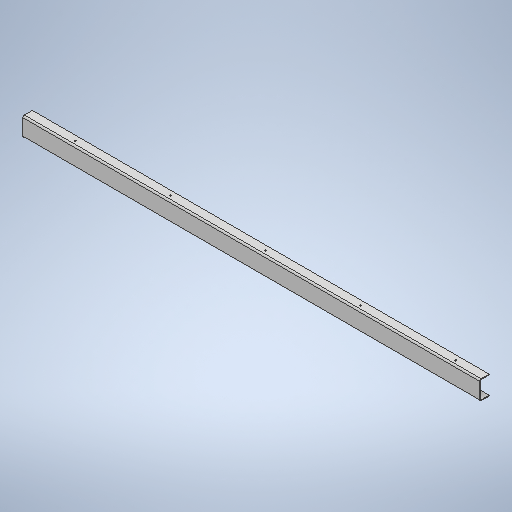
# Autodesk Inventor part: B_Beam
Saved by Autodesk Inventor 2025.2 (Build 292293000, 293)
## iProperties
Created: 2025-04-01
Part Number: B_Beam
Material: Generic
Document SubType Name: Sheet Metal
Designer: Caspe
Density: 1 g/cm^3
Sheet Metal Rule: Default_mm
Appearance: Default
Author: Caspe
Autodesk Inventor part; units mm, degrees
ref_plane "YZ Plane" through (0, 0, 0) normal (1, 0, 0) x (0, 1, 0)
ref_plane "XZ Plane" through (0, 0, 0) normal (0, 1, 0) x (-1, 0, 0)
ref_plane "XY Plane" through (0, 0, 0) normal (0, 0, 1) x (1, 0, 0)
sketch "Sketch2" plane through (0, 0, 0) normal (0, 0, 1) x (-1, 0, 0)
  line L0 (0, 0) -> (-1200, 0)
  line L1 (-1200, 0) -> (-1200, -50)
  line L2 (-1200, -50) -> (0, -50)
  line L3 (0, -50) -> (0, 0)
  dimension "d2" = 1200
  dimension "d3" = 50
  measures "d2" distance of L2.end L1.end
  measures "d3" distance of L1.end L0.end
extrude "Plate1" add sketch "Sketch2" along normal blind 2
sketch "Sketch3" plane through (1200, 48, 2) normal (0, 1, 0) x (-1, 0, 0)
  line L0 (1200, 0) -> (0, 0)
  line L1 (0, 0) -> (0, -25)
  line L2 (0, -25) -> (1200, -25)
  line L3 (1200, -25) -> (1200, 0)
  constraints: 6 end point, 1 horizontal, 1 perpendicular, 1 vertical
edge flange "Flange1" height 25 angle 90 thickness 2 bend radius 2 thickness toward (0, 1, 0) relief straight relief width 2 relief depth 1 corner gap 2 corner form 0 edges at (600, 50, 0) (600, 0, 0) wall of the first edge with corners at (0, 48, 2) (1200, 48, 2) (1200, 48, -23) (0, 48, -23)
bend "Bend1"
corner "Corner1"
sketch "Sketch4" plane through (0, 50, -23) normal (0, 1, 0) x (1, 0, 0)
  circle A0 centre (125, -12.5) radius 2
  line L0 (1200, -25) -> (0, -25) projected
  line L1 (0, -21) -> (0, 0) projected
  circle A1 centre (375, -12.5) radius 2
  circle A2 centre (625, -12.5) radius 2
  circle A3 centre (875, -12.5) radius 2
  circle A4 centre (1125, -12.5) radius 2
  point P0 (0, -23)
  dimension "d15" = 4
  dimension "d16" = 12.5
  dimension "d17" = 125
  dimension "d20" = 250
  constraints: 5 centre point, 1 horizontal, 8 other
  measures "d15" diameter of A0
  measures "d16" distance from line of L0 A0.centre
  measures "d17" distance from line of L1 A0.centre
  measures "d20" distance of A0.centre A1.centre
extrude "Cut1" cut sketch "Sketch4" against normal up to surface (50 mm away)
equation "\"d2\" = B_length"
equation "\"d3\" = B_width"
equation "\"d15\" = rivet_diameter"
equation "\"d16\" = 0.25 * B_width"
equation "\"d17\" = 0.5 * rivet_displacement"
equation "\"d20\" = rivet_displacement"
equation "\"d25\" = Thickness"
equation "\"d4\" = Thickness"
equation "\"d5\" = BendReliefWidth"
equation "\"d6\" = BendReliefDepth"
equation "\"d7\" = MinimumRemnant"
equation "\"d8\" = TransitionRadius"
equation "\"d9\" = 0.5 * B_width"
equation "\"d11\" = BendRadius"
equation "\"d12\" = CornerReliefSize"
equation "\"d13\" = GapSize"
equation "\"d14\" = JacobiRadiusSize"
equation "\"Thickness\" = plate_thickness"
equation "\"BendRadius\" = Thickness"
equation "\"BendReliefWidth\" = Thickness"
equation "\"BendReliefDepth\" = 0.5 * Thickness"
equation "\"CornerReliefSize\" = 4 * Thickness"
equation "\"MinimumRemnant\" = 2 * Thickness"
equation "\"TransitionRadius\" = BendRadius"
equation "\"JacobiRadiusSize\" = BendRadius"
equation "\"GapSize\" = Thickness"
equation "\"A_joint_tolerance\" = 3"
equation "\"l___________\" = 0"
equation "\"B_length\" = 1200"
equation "\"B_width\" = 50"
equation "\"l__________\" = 0"
equation "\"l_________\" = 0"
equation "\"rivet_diameter\" = 4"
equation "\"rivet_displacement\" = 250"
equation "\"plate_thickness\" = 2"
equation "\"l________\" = 0"
body "Solid1"
